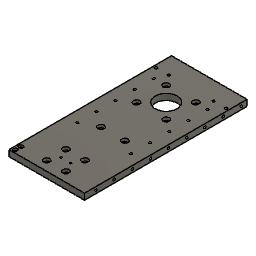
Z-AxisAssy v53 (Autodesk Fusion 360 archive; units mm, degrees)
design "PlaceHeadPlate" references "tormach 770mx"
Autodesk Fusion 360 part; units mm, degrees
sketch "Sketch1" plane through (0, 0, 0) normal (0, 1, 0) x (1, 0, 0)
  line L0 (0, 0) -> (79, 0)
  line L1 (79, 0) -> (79, -170)
  line L2 (79, -170) -> (0, -170)
  line L3 (0, -170) -> (0, 0)
  line L4 (39.5, 0) -> (39.5, -169.9926) construction
  line L5 (49.5, -160) -> (29.5, -160) construction
  line L6 (29.5, -160) -> (29.5, -140) construction
  line L7 (29.5, -140) -> (49.5, -140) construction
  line L8 (49.5, -140) -> (49.5, -160) construction
  line L9 (49.5, -160) -> (29.5, -140) construction
  line L10 (29.5, -160) -> (49.5, -140) construction
  line L11 (55, -60.5) -> (24, -60.5) construction
  line L12 (24, -60.5) -> (24, -29.5) construction
  line L13 (24, -29.5) -> (55, -29.5) construction
  line L14 (55, -29.5) -> (55, -60.5) construction
  line L15 (55, -60.5) -> (24, -29.5) construction
  line L16 (24, -60.5) -> (55, -29.5) construction
  circle A0 centre (39.5, -45) radius 11.5
  point P0 (67.5, -110)
  point P1 (11.5, -110)
  point P2 (67.5, -90)
  point P3 (11.5, -90)
  point P4 (67.5, -70)
  point P5 (11.5, -70)
  point P6 (67.5, -50)
  point P7 (11.5, -50)
  point P8 (67.5, -30)
  point P9 (11.5, -30)
  point P10 (39.5, -150)
  point P11 (29.5, -140)
  point P12 (49.5, -140)
  point P13 (49.5, -160)
  point P14 (29.5, -160)
  point P15 (44.5, -150)
  point P16 (34.5, -150)
  point P17 (3.5, -167)
  point P18 (3.5, -161)
  point P19 (27.58, -101.35)
  point P20 (52.58, -101.35)
  point P21 (39.5, -45)
  point P22 (24, -29.5)
  point P23 (55, -29.5)
  point P24 (55, -60.5)
  point P25 (24, -60.5)
  point P26 (16, -19)
  point P27 (63, -19)
  point P28 (2.86, -19)
  point P29 (76.14, -19)
  dimension "d1" = 79
  dimension "d2" = 170
  dimension "d5" = 60
  dimension "d6" = 11.5
  dimension "d7" = 56
  dimension "d10" = 0
  dimension "d11" = 20
  dimension "d15" = 20
  dimension "d16" = 20
  dimension "d17" = 10
  dimension "d18" = 10
  dimension "d19" = 5
  dimension "d20" = 6
  dimension "d21" = 3.5
  dimension "d22" = 3
  dimension "d23" = 25
  dimension "d24" = 68.65
  dimension "d25" = 11.92
  dimension "d26" = 31
  dimension "d27" = 31
  dimension "d28" = 29.5
  dimension "d29" = 24
  dimension "d31" = 16
  dimension "d32" = 16
  dimension "d33" = 19
  dimension "d34" = 13.14
  dimension "d35" = 13.14
  dimension "d36" = 19
  dimension "d42" = 23
  constraint horizontal L0
  constraint vertical L1
  constraint horizontal L2
  constraint vertical L3
  constraint coincident L0.start L3.end
  constraint horizontal P0 P1
  constraint perpendicular L2 L4
  constraint horizontal L5
  constraint perpendicular L5 L6
  constraint parallel L5 L7
  constraint parallel L6 L8
  constraint coincident L9 P10
  constraint coincident L10 P10
  constraint coincident L4 P10
  constraint coincident P11 L6.end
  constraint coincident P12 L7.end
  constraint coincident P13 L5.start
  constraint coincident P14 L5.end
  constraint horizontal P15 P16
  constraint vertical P17 P18
  constraint horizontal P19 P20
  constraint horizontal L11
  constraint perpendicular L11 L12
  constraint parallel L11 L13
  constraint parallel L12 L14
  constraint coincident L15 P21
  constraint coincident L16 P21
  constraint coincident L4 P21
  constraint coincident P22 L12.end
  constraint coincident P23 L13.end
  constraint coincident P24 L11.start
  constraint coincident P25 L11.end
  constraint horizontal P26 P27
  constraint horizontal P28 P29
  constraint coincident P21 A0.centre
  measures "d1" distance of L0.start L0.end
  measures "d2" distance of L0.start L2.end
  measures "d5" distance of L2 P0
  measures "d6" distance of L1 P0
  measures "d7" distance of P0 P1
  measures "d15" distance of P11 P12
  measures "d16" distance of L5 L7
  measures "d17" distance of L2 L5
  measures "d18" distance of P15 P16
  measures "d19" distance of L8 P15
  measures "d20" distance of P17 P18
  measures "d21" distance of L3 P17
  measures "d22" distance of L2 P17
  measures "d23" distance of P19 P20
  measures "d24" distance of L2 P19
  measures "d25" distance of L4 P19
  measures "d26" distance of P22 P23
  measures "d27" distance of P25 P22
  measures "d28" distance of L0 L13
  measures "d29" distance of L3 L12
  measures "d31" distance of L3 P26
  measures "d32" distance of L1 P27
  measures "d33" distance of L0 P26
  measures "d34" horizontal distance of P26 P28
  measures "d35" horizontal distance of P27 P29
  measures "d36" distance of L0 P28
  measures "d42" diameter of A0
extrude "Extrude2" add sketch "Sketch1" against normal blind 6.41
hole "Hole2" at (3.5, 0, 161) direction (0, -1, 0) diameter 2 end through all counterbore diameter 4.4 counterbore depth 2
hole "Hole3" at (3.5, 0, 167) direction (0, -1, 0) diameter 2 end through all counterbore diameter 4.4 counterbore depth 2
sketch "Sketch2" plane through (0, -6.41, 0) normal (0, -1, 0) x (1, 0, 0)
  circle A0 centre (3.5, 167) radius 1
  circle A1 centre (3.5, 161) radius 1
  circle A2 centre (39.5, 45) radius 11.5
  line L0 (79, 170) -> (0, 170)
  line L1 (0, 170) -> (0, 0)
  line L2 (0, 0) -> (79, 0)
  line L3 (79, 0) -> (79, 170)
  line L4 (49.5, 140) -> (49.5, 160)
  point P0 (44.5, 150)
  point P1 (34.5, 150)
  dimension "d55" = 5
  dimension "d56" = 10
  constraint horizontal P0 P1
  measures "d55" distance of P0 L4
  measures "d56" distance of P0 P1
hole "Hole4" at (34.5, -6.41, 150) direction (0, 1, 0) diameter 2 end through all counterbore diameter 4.4 counterbore depth 2
hole "Hole5" at (44.5, -6.41, 150) direction (0, 1, 0) diameter 2 end through all counterbore diameter 4.4 counterbore depth 2
hole "Hole6" at (29.5, 0, 140) direction (0, -1, 0) diameter 3.4 end through all counterbore diameter 6.5 counterbore depth 3
hole "Hole7" at (49.5, 0, 140) direction (0, -1, 0) diameter 3.4 end through all counterbore diameter 6.5 counterbore depth 3
hole "Hole8" at (29.5, 0, 160) direction (0, -1, 0) diameter 3.4 end through all counterbore diameter 6.5 counterbore depth 3
hole "Hole9" at (49.5, 0, 160) direction (0, -1, 0) diameter 3.4 end through all counterbore diameter 6.5 counterbore depth 3
hole "Hole10" at (27.58, 0, 101.35) direction (0, -1, 0) diameter 3.4 end through all counterbore diameter 6.5 counterbore depth 3
hole "Hole11" at (52.58, 0, 101.35) direction (0, -1, 0) diameter 3.4 end through all counterbore diameter 6.5 counterbore depth 3
hole "Hole12" at (24, 0, 29.5) direction (0, -1, 0) diameter 3.4 end through all counterbore diameter 6.5 counterbore depth 3
hole "Hole13" at (55, 0, 29.5) direction (0, -1, 0) diameter 3.4 end through all counterbore diameter 6.5 counterbore depth 3
hole "Hole14" at (55, 0, 60.5) direction (0, -1, 0) diameter 3.4 end through all counterbore diameter 6.5 counterbore depth 3
hole "Hole15" at (24, 0, 60.5) direction (0, -1, 0) diameter 3.4 end through all counterbore diameter 6.5 counterbore depth 3
hole "Hole16" at (11.5, 0, 110) direction (0, -1, 0) diameter 2.5 end through all
hole "Hole17" at (11.5, 0, 90) direction (0, -1, 0) diameter 2.5 end through all
hole "Hole18" at (11.5, 0, 70) direction (0, -1, 0) diameter 2.5 end through all
hole "Hole19" at (11.5, 0, 50) direction (0, -1, 0) diameter 2.5 end through all
hole "Hole20" at (11.5, 0, 30) direction (0, -1, 0) diameter 2.5 end through all
hole "Hole21" at (67.5, 0, 110) direction (0, -1, 0) diameter 2.5 end through all
hole "Hole22" at (67.5, 0, 90) direction (0, -1, 0) diameter 2.5 end through all
hole "Hole23" at (67.5, 0, 70) direction (0, -1, 0) diameter 2.5 end through all
hole "Hole24" at (67.5, 0, 50) direction (0, -1, 0) diameter 2.5 end through all
hole "Hole25" at (67.5, 0, 30) direction (0, -1, 0) diameter 2.5 end through all
hole "Hole26" at (16, 0, 19) direction (0, -1, 0) diameter 2.5 end through all
hole "Hole27" at (63, 0, 19) direction (0, -1, 0) diameter 2.5 end through all
hole "Hole28" at (2.86, 0, 19) direction (0, -1, 0) diameter 2.8 end through all
hole "Hole29" at (76.14, 0, 19) direction (0, -1, 0) diameter 2.8 end through all
sketch "TopHolesSketch" plane through (0, 0, 0) normal (0, 0, -1) x (-1, 0, 0)
  line L0 (0, 0) -> (-79, 0)
  line L1 (-79, 0) -> (-79, -6.41)
  line L2 (-79, -6.41) -> (0, -6.41)
  line L3 (0, -6.41) -> (0, 0)
  line L4 (0, -3.205) -> (-79, -3.205) construction
  point P0 (-14, -3.205)
  point P1 (-31, -3.205)
  point P2 (-48, -3.205)
  point P3 (-65, -3.205)
  dimension "d159" = 14
  dimension "d162" = -17
  dimension "d163" = 0
  constraint midpoint L3 L4.start
  constraint midpoint L1 L4.end
  constraint coincident L4 P0
  measures "d159" distance of L3 P0
hole "Hole30" at (14, -3.205, 0) direction (0, 0, 1) diameter 2.5 depth 10 tip angle 118
pattern_linear "R-Pattern1" count 4 spacing 17 along (1, 0, 0) of "Hole30"
sketch "Sketch4" plane through (0, 0, 0) normal (-1, 0, 0) x (0, 0, 1)
  line L0 (170, 0) -> (0, 0)
  line L1 (0, 0) -> (0, -6.41)
  line L2 (0, -6.41) -> (170, -6.41)
  line L3 (170, -6.41) -> (170, 0)
  line L4 (0, -3.205) -> (170, -3.205) construction
  point P0 (6, -3.205)
  point P1 (25, -3.205)
  point P2 (44, -3.205)
  point P3 (63, -3.205)
  point P4 (82, -3.205)
  point P5 (101, -3.205)
  point P6 (120, -3.205)
  point P7 (139, -3.205)
  point P8 (158, -3.205)
  dimension "d171" = 6
  dimension "d174" = 19
  dimension "d175" = 0
  constraint midpoint L1 L4.start
  constraint midpoint L3 L4.end
  constraint coincident L4 P0
  measures "d171" distance of L1 P0
sketch "Sketch5" plane through (79, 0, 0) normal (1, 0, 0) x (0, 0, -1)
  line L0 (0, 0) -> (-170, 0)
  line L1 (-170, 0) -> (-170, -6.41)
  line L2 (-170, -6.41) -> (0, -6.41)
  line L3 (0, -6.41) -> (0, 0)
  line L4 (0, -3.205) -> (-170, -3.205) construction
  point P0 (-6, -3.205)
  point P1 (-25, -3.205)
  point P2 (-44, -3.205)
  point P3 (-63, -3.205)
  point P4 (-82, -3.205)
  point P5 (-101, -3.205)
  point P6 (-120, -3.205)
  point P7 (-139, -3.205)
  point P8 (-158, -3.205)
  dimension "d176" = 6
  dimension "d179" = -19
  dimension "d180" = 0
  constraint midpoint L3 L4.start
  constraint midpoint L1 L4.end
  constraint coincident L4 P0
  measures "d176" distance of L3 P0
hole "Hole31" at (79, -3.205, 6) direction (-1, 0, 0) diameter 2.5 depth 10 tip angle 118
pattern_linear "R-Pattern2" count 1 spacing 19 along (0, -1, 0) count 9 spacing 19 along (0, 0, 1) of "Hole31"
hole "Hole32" at (0, -3.205, 6) direction (1, 0, 0) diameter 2.5 depth 10 tip angle 118
pattern_linear "R-Pattern3" count 1 spacing 0 along (0, -1, 0) count 9 spacing 19 along (0, 0, 1) of "Hole32"

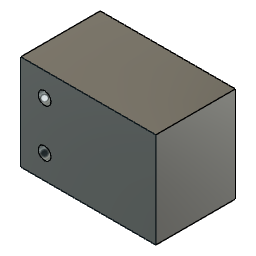
design "X-AxisLimitSwitchBlock"
Autodesk Fusion 360 part; units mm, degrees
sketch "Sketch1" plane through (0, 0, 0) normal (0, 1, 0) x (1, 0, 0)
  line L0 (0, 0) -> (17, 0)
  line L1 (17, 0) -> (17, -10)
  line L2 (17, -10) -> (0, -10)
  line L3 (0, -10) -> (0, 0)
  dimension "d1" = 17
  dimension "d2" = 10
  constraint horizontal L0
  constraint vertical L1
  constraint horizontal L2
  constraint vertical L3
  constraint coincident L0.start L3.end
  measures "d1" distance of L0.start L0.end
  measures "d2" distance of L0.start L2.end
extrude "Extrude1" add sketch "Sketch1" along normal blind 12
sketch "Sketch2" plane through (0, 0, 10) normal (0, 0, 1) x (1, 0, 0)
  line L0 (0, 0) -> (17, 0)
  line L1 (17, 0) -> (17, 12)
  line L2 (17, 12) -> (0, 12)
  line L3 (0, 12) -> (0, 0)
  point P0 (3, 3)
  point P1 (3, 9)
  dimension "d5" = 3
  dimension "d6" = 3
  dimension "d7" = 6
  measures "d5" distance of L0 P0
  measures "d6" distance of L3 P0
  measures "d7" distance of P0 P1
hole "Hole1" at (3, 3, 10) direction (0, 0, -1) diameter 1.6 depth 5 tip angle 118
hole "Hole2" at (3, 9, 10) direction (0, 0, -1) diameter 1.6 depth 5 tip angle 118

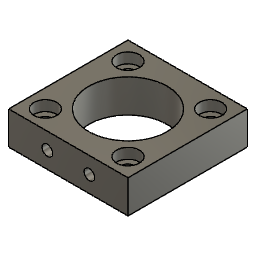
design "Nema8Mount" references "tormach 770mx"
Autodesk Fusion 360 part; units mm, degrees
sketch "Sketch1" plane through (0, 0, 0) normal (0, 1, 0) x (1, 0, 0)
  line L0 (11.55, -11.55) -> (-11.55, -11.55)
  line L1 (-11.55, -11.55) -> (-11.55, 11.55)
  line L2 (-11.55, 11.55) -> (11.55, 11.55)
  line L3 (11.55, 11.55) -> (11.55, -11.55)
  line L4 (11.55, -11.55) -> (-11.55, 11.55) construction
  line L5 (-11.55, -11.55) -> (11.55, 11.55) construction
  dimension "d1" = 23.1
  dimension "d2" = 23.1
  constraint horizontal L0
  constraint perpendicular L0 L1
  constraint parallel L0 L2
  constraint parallel L1 L3
  constraint coincident L4 origin
  constraint coincident L5 origin
  measures "d1" distance of L1.end L2.end
  measures "d2" distance of L0.end L1.end
extrude "Extrude1" add sketch "Sketch1" along normal blind 6.4
sketch "Sketch2" plane through (0, 6.4, 0) normal (0, 1, 0) x (-1, 0, 0)
  line L0 (-11.55, -11.55) -> (11.55, -11.55)
  line L1 (11.55, -11.55) -> (11.55, 11.55)
  line L2 (11.55, 11.55) -> (-11.55, 11.55)
  line L3 (-11.55, 11.55) -> (-11.55, -11.55)
  line L4 (-8, 8) -> (8, 8) construction
  line L5 (8, 8) -> (8, -8) construction
  line L6 (8, -8) -> (-8, -8) construction
  line L7 (-8, -8) -> (-8, 8) construction
  line L8 (-8, 8) -> (8, -8) construction
  line L9 (8, 8) -> (-8, -8) construction
  circle A0 centre (0, 0) radius 7.6
  point P0 (8, -8)
  point P1 (-8, -8)
  point P2 (-8, 8)
  point P3 (8, 8)
  dimension "d5" = 16
  dimension "d6" = 16
  dimension "d7" = 15.2
  constraint horizontal L4
  constraint perpendicular L4 L5
  constraint parallel L4 L6
  constraint parallel L5 L7
  constraint coincident L8 A0.centre
  constraint coincident L9 A0.centre
  constraint coincident A0.centre origin
  constraint coincident P0 L5.end
  constraint coincident P1 L6.end
  constraint coincident P2 L4.start
  constraint coincident P3 L4.end
  measures "d5" distance of P0 P1
  measures "d6" distance of P3 P0
  measures "d7" diameter of A0
hole "Hole1" at (-8, 6.4, -8) direction (0, -1, 0) diameter 2.2 end through all counterbore diameter 4.4 counterbore depth 2
hole "Hole2" at (8, 6.4, -8) direction (0, -1, 0) diameter 2.2 end through all counterbore diameter 4.4 counterbore depth 2
hole "Hole3" at (8, 6.4, 8) direction (0, -1, 0) diameter 2.2 end through all counterbore diameter 4.4 counterbore depth 2
hole "Hole4" at (-8, 6.4, 8) direction (0, -1, 0) diameter 2.2 end through all counterbore diameter 4.4 counterbore depth 2
extrude "Extrude2" cut sketch "Sketch2" along normal through all and the other way through all contours A0
sketch "Sketch3" plane through (0, 0, 11.55) normal (0, 0, 1) x (1, 0, 0)
  line L0 (-11.55, 0) -> (11.55, 0)
  line L1 (11.55, 0) -> (11.55, 6.4)
  line L2 (11.55, 6.4) -> (-11.55, 6.4)
  line L3 (-11.55, 6.4) -> (-11.55, 0)
  line L4 (-11.55, 3.2) -> (11.55, 3.2) construction
  point P0 (-4.15, 3.2)
  point P1 (3.99, 3.2)
  dimension "d29" = 8.14
  dimension "d30" = 7.4
  constraint midpoint L3 L4.start
  constraint midpoint L1 L4.end
  constraint coincident L4 P0
  constraint coincident L4 P1
  measures "d29" distance of P0 P1
  measures "d30" distance of L3 P0
hole "Hole5" at (-4.07, 3.2, 11.55) direction (0, 0, -1) diameter 2.05 depth 7 tip angle 118
hole "Hole6" at (4.07, 3.2, 11.55) direction (0, 0, -1) diameter 2.05 depth 7 tip angle 118

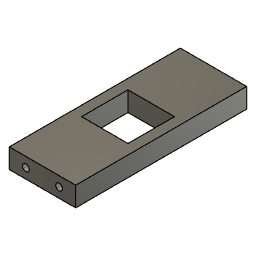
design "CameraHolder" references "tormach 770mx"
Autodesk Fusion 360 part; units mm, degrees
sketch "Sketch1" plane through (0, 0, 0) normal (0, 1, 0) x (1, 0, 0)
  line L0 (0, 0) -> (20, 0)
  line L1 (20, 0) -> (20, -51.54)
  line L2 (20, -51.54) -> (0, -51.54)
  line L3 (0, -51.54) -> (0, 0)
  dimension "d1" = 20
  dimension "d2" = 51.54
  constraint horizontal L0
  constraint vertical L1
  constraint horizontal L2
  constraint vertical L3
  constraint coincident L0.start L3.end
  measures "d1" distance of L0.start L0.end
  measures "d2" distance of L0.start L2.end
extrude "Extrude1" add sketch "Sketch1" along normal blind 5.92
sketch "Sketch2" plane through (0, 5.92, 0) normal (0, 1, 0) x (-1, 0, 0)
  line L0 (0, 51.54) -> (-20, 51.54)
  line L1 (-20, 51.54) -> (-20, 0)
  line L2 (-20, 0) -> (0, 0)
  line L3 (0, 0) -> (0, 51.54)
  line L4 (-10, 0) -> (-10, 49) construction
  line L5 (0, 25.77) -> (-20, 25.77) construction
  line L6 (-3, 32.77) -> (-17, 32.77)
  line L7 (-17, 32.77) -> (-17, 18.77)
  line L8 (-17, 18.77) -> (-3, 18.77)
  line L9 (-3, 18.77) -> (-3, 32.77)
  line L10 (-3, 32.77) -> (-17, 18.77) construction
  line L11 (-17, 32.77) -> (-3, 18.77) construction
  point P0 (-10, 25.77)
  dimension "d5" = 14
  dimension "d6" = 14
  constraint midpoint L2 L4.start
  constraint perpendicular L2 L4
  constraint midpoint L3 L5.start
  constraint midpoint L1 L5.end
  constraint horizontal L6
  constraint perpendicular L6 L7
  constraint parallel L6 L8
  constraint parallel L7 L9
  constraint coincident L10 P0
  constraint coincident L11 P0
  constraint midpoint L5 P0
  constraint coincident L9.start L8
  constraint coincident L8.end L9
  constraint coincident L7.end L8
  constraint coincident L8.start L7
  constraint coincident L6.start L9
  constraint coincident L9.end L6
  constraint coincident L6.end L7
  constraint coincident L7.start L6
  measures "d5" distance of L7.end L8.end
  measures "d6" distance of L6.end L7.end
extrude "Extrude2" cut sketch "Sketch2" along normal through all and the other way through all contours L6 L7 L8 L9
sketch "Sketch3" plane through (0, 0, 51.54) normal (0, 0, 1) x (1, 0, 0)
  line L0 (0, 0) -> (20, 0)
  line L1 (20, 0) -> (20, 5.92)
  line L2 (20, 5.92) -> (0, 5.92)
  line L3 (0, 5.92) -> (0, 0)
  line L4 (10, 5.92) -> (10, 0) construction
  line L5 (20, 2.96) -> (0, 2.96) construction
  point P0 (5, 2.96)
  point P1 (15, 2.96)
  dimension "d12" = 10
  dimension "d13" = 5
  constraint midpoint L2 L4.start
  constraint midpoint L0 L4.end
  constraint midpoint L1 L5.start
  constraint midpoint L3 L5.end
  constraint coincident L5 P0
  constraint coincident L5 P1
  measures "d12" distance of P0 P1
  measures "d13" distance of L5.end P0
hole "Hole1" at (5, 2.96, 51.54) direction (0, 0, -1) diameter 2.05 depth 10 tip angle 118
hole "Hole2" at (15, 2.96, 51.54) direction (0, 0, -1) diameter 2.05 depth 10 tip angle 118
sketch "Sketch4" plane through (0, 0, 0) normal (0, 0, -1) x (-1, 0, 0)
  line L0 (-20, 0) -> (0, 0)
  line L1 (0, 0) -> (0, 5.92)
  line L2 (0, 5.92) -> (-20, 5.92)
  line L3 (-20, 5.92) -> (-20, 0)
  line L4 (-20, 2.96) -> (0, 2.96) construction
  point P0 (-15, 2.96)
  point P1 (-5, 2.96)
  dimension "d30" = 10
  dimension "d31" = 5
  constraint midpoint L3 L4.start
  constraint midpoint L1 L4.end
  constraint coincident L4 P0
  constraint coincident L4 P1
  measures "d30" distance of P0 P1
  measures "d31" distance of L3 P0
hole "Hole5" at (15, 2.96, 0) direction (0, 0, 1) diameter 2.05 depth 10 tip angle 118
hole "Hole6" at (5, 2.96, 0) direction (0, 0, 1) diameter 2.05 depth 10 tip angle 118

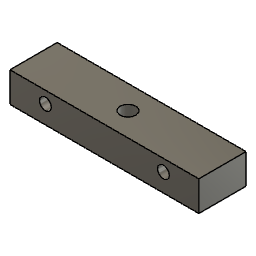
design "CableClampBracket" references "tormach 770mx"
Autodesk Fusion 360 part; units mm, degrees
sketch "Sketch1" plane through (0, 0, 0) normal (0, 1, 0) x (1, 0, 0)
  line L0 (0, 0) -> (40, 0)
  line L1 (40, 0) -> (40, -10)
  line L2 (40, -10) -> (0, -10)
  line L3 (0, -10) -> (0, 0)
  dimension "d1" = 40
  dimension "d2" = 10
  constraint horizontal L0
  constraint vertical L1
  constraint horizontal L2
  constraint vertical L3
  constraint coincident L0.start L3.end
  measures "d1" distance of L0.start L0.end
  measures "d2" distance of L0.start L2.end
extrude "Extrude1" add sketch "Sketch1" along normal blind 6.35
sketch "Sketch2" plane through (0, 6.35, 0) normal (0, 1, 0) x (-1, 0, 0)
  line L0 (0, 10) -> (-40, 10)
  line L1 (-40, 10) -> (-40, 0)
  line L2 (-40, 0) -> (0, 0)
  line L3 (0, 0) -> (0, 10)
  line L4 (0, 5) -> (-40, 5) construction
  point P0 (-20, 5)
  constraint midpoint L3 L4.start
  constraint midpoint L1 L4.end
  constraint midpoint L4 P0
hole "Hole1" at (20, 6.35, 5) direction (0, -1, 0) diameter 3.3 end through all
sketch "Sketch3" plane through (0, 0, 10) normal (0, 0, 1) x (1, 0, 0)
  line L0 (0, 0) -> (40, 0)
  line L1 (40, 0) -> (40, 6.35)
  line L2 (40, 6.35) -> (0, 6.35)
  line L3 (0, 6.35) -> (0, 0)
  line L4 (0, 3.85) -> (39.5878, 3.85) construction
  point P0 (7.5, 3.85)
  point P1 (32.5, 3.85)
  dimension "d10" = 7.5
  dimension "d11" = 25
  dimension "d18" = 2.5
  constraint coincident L4 P0
  constraint coincident L4 P1
  measures "d10" distance of L3 P0
  measures "d11" distance of P0 P1
  measures "d18" distance of L2 L4
hole "Hole4" at (7.5, 3.85, 10) direction (0, 0, -1) diameter 2.5 end through all
hole "Hole5" at (32.5, 3.85, 10) direction (0, 0, -1) diameter 2.5 end through all
hole "Hole2" [suppressed]
hole "Hole3" [suppressed]

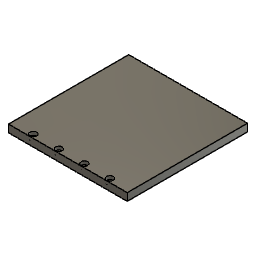
design "PlaceHeadCover"
Autodesk Fusion 360 part; units mm, degrees
sketch "Sketch1" plane through (0, 0, 0) normal (0, 1, 0) x (1, 0, 0)
  line L0 (0, 0) -> (79, 0)
  line L1 (79, 0) -> (79, -80)
  line L2 (79, -80) -> (0, -80)
  line L3 (0, -80) -> (0, 0)
  dimension "d1" = 79
  dimension "d2" = 80
  constraint horizontal L0
  constraint vertical L1
  constraint horizontal L2
  constraint vertical L3
  constraint coincident L0.start L3.end
  measures "d1" distance of L0.start L0.end
  measures "d2" distance of L0.start L2.end
extrude "Extrude1" add sketch "Sketch1" along normal blind 5
sketch "Sketch2" plane through (0, 5, 0) normal (0, 1, 0) x (-1, 0, 0)
  line L0 (0, 80) -> (-79, 80)
  line L1 (-79, 80) -> (-79, 0)
  line L2 (-79, 0) -> (0, 0)
  line L3 (0, 0) -> (0, 80)
  point P0 (-14, 77.5)
  dimension "d5" = 14
  dimension "d6" = 2.5
  measures "d5" distance of L3 P0
  measures "d6" distance of L0 P0
hole "Hole1" at (14, 5, 77.5) direction (0, -1, 0) diameter 2 end through all counterbore diameter 4.4 counterbore depth 2.2
pattern_linear "R-Pattern1" count 1 spacing 0 along (0, 0, -1) count 4 spacing 17 along (1, 0, 0) of "Hole1"

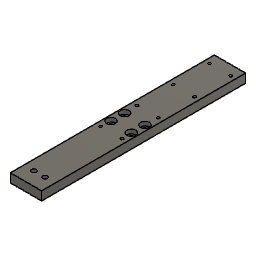
design "Z-AxisGearRackPlateFixed" references "tormach 770mx"
Autodesk Fusion 360 part; units mm, degrees
sketch "Sketch1" plane through (0, 0, 0) normal (0, 1, 0) x (1, 0, 0)
  line L0 (0, 0) -> (23, 0)
  line L1 (23, 0) -> (23, -150)
  line L2 (23, -150) -> (0, -150)
  line L3 (0, -150) -> (0, 0)
  dimension "d1" = 23
  dimension "d2" = 150
  constraint horizontal L0
  constraint vertical L1
  constraint horizontal L2
  constraint vertical L3
  constraint coincident L0.start L3.end
  measures "d1" distance of L0.start L0.end
  measures "d2" distance of L0.start L2.end
extrude "Extrude1" add sketch "Sketch1" along normal blind 6.43
sketch "Sketch2" plane through (0, 6.43, 0) normal (0, 1, 0) x (1, 0, 0)
  line L0 (11.5, 0) -> (11.5, -150) construction
  line L1 (0, 0) -> (0, -150)
  line L2 (0, -75) -> (23, -75) construction
  line L3 (19, -70) -> (4, -70) construction
  line L4 (4, -70) -> (4, -80) construction
  line L5 (4, -80) -> (19, -80) construction
  line L6 (19, -80) -> (19, -70) construction
  line L7 (19, -70) -> (4, -80) construction
  line L8 (4, -70) -> (19, -80) construction
  line L9 (23, 0) -> (0, 0)
  line L10 (0, -150) -> (23, -150)
  line L11 (0, -150) -> (23, -150)
  line L12 (23, -150) -> (23, 0)
  line L13 (23, 0) -> (0, 0)
  line L14 (0, 0) -> (0, -150)
  point P0 (11.5, -75)
  point P1 (4, -70)
  point P2 (19, -70)
  point P3 (19, -80)
  point P4 (4, -80)
  point P5 (3.7, -7.25)
  point P6 (19.3, -7.25)
  point P7 (3.7, -33.92)
  point P8 (3.7, -60.59)
  point P9 (3.7, -87.26)
  point P10 (19.3, -33.92)
  point P11 (19.3, -60.59)
  point P12 (19.3, -87.26)
  dimension "d5" = 11.5
  dimension "d6" = 15
  dimension "d7" = 10
  dimension "d8" = 15.6
  dimension "d9" = 19.3
  dimension "d10" = 7.25
  dimension "d13" = 0
  dimension "d14" = -26.67
  dimension "d17" = 0
  dimension "d18" = -26.67
  constraint vertical L0
  constraint midpoint L1 L2.start
  constraint perpendicular L0 L2
  constraint horizontal L3
  constraint perpendicular L3 L4
  constraint parallel L3 L5
  constraint parallel L4 L6
  constraint coincident L7 P0
  constraint coincident L8 P0
  constraint midpoint L0 P0
  constraint coincident P1 L3.end
  constraint coincident P2 L3.start
  constraint coincident P3 L5.end
  constraint coincident P4 L4.end
  constraint horizontal P5 P6
  measures "d5" distance of L0 L1
  measures "d6" distance of P4 P3
  measures "d7" distance of P1 P4
  measures "d8" distance of P5 P6
  measures "d9" distance of L1 P6
  measures "d10" distance of P5 L9
hole "Hole1" at (4, 6.43, 70) direction (0, -1, 0) diameter 3.4 end through all counterbore diameter 6.5 counterbore depth 3
hole "Hole2" at (19, 6.43, 70) direction (0, -1, 0) diameter 3.4 end through all counterbore diameter 6.5 counterbore depth 3
hole "Hole3" at (4, 6.43, 80) direction (0, -1, 0) diameter 3.4 end through all counterbore diameter 6.5 counterbore depth 3
hole "Hole4" at (19, 6.43, 80) direction (0, -1, 0) diameter 3.4 end through all counterbore diameter 6.5 counterbore depth 3
hole "Hole5" at (3.7, 6.43, 7.25) direction (0, -1, 0) diameter 2.05 end through all
hole "Hole6" at (19.3, 6.43, 7.25) direction (0, -1, 0) diameter 2.05 end through all
hole "Hole7" at (3.7, 6.43, 33.92) direction (0, -1, 0) diameter 2.05 end through all
hole "Hole8" at (19.3, 6.43, 33.92) direction (0, -1, 0) diameter 2.05 end through all
hole "Hole9" at (3.7, 6.43, 60.59) direction (0, -1, 0) diameter 2.05 end through all
hole "Hole10" at (19.3, 6.43, 60.59) direction (0, -1, 0) diameter 2.05 end through all
hole "Hole11" at (3.7, 6.43, 87.26) direction (0, -1, 0) diameter 2.05 end through all
hole "Hole12" at (19.3, 6.43, 87.26) direction (0, -1, 0) diameter 2.05 end through all
sketch "Sketch3" plane through (0, 0, 0) normal (0, -1, 0) x (1, 0, 0)
  circle A0 centre (19.3, 87.26) radius 1.025
  circle A1 centre (3.7, 87.26) radius 1.025
  circle A2 centre (19.3, 60.59) radius 1.025
  circle A3 centre (3.7, 60.59) radius 1.025
  circle A4 centre (19.3, 33.92) radius 1.025
  circle A5 centre (3.7, 33.92) radius 1.025
  circle A6 centre (19.3, 7.25) radius 1.025
  circle A7 centre (3.7, 7.25) radius 1.025
  circle A8 centre (19, 80) radius 1.7
  circle A9 centre (4, 80) radius 1.7
  circle A10 centre (19, 70) radius 1.7
  circle A11 centre (4, 70) radius 1.7
  line L0 (23, 150) -> (0, 150)
  line L1 (0, 150) -> (0, 0)
  line L2 (0, 0) -> (23, 0)
  line L3 (23, 0) -> (23, 150)
  line L4 (0, 150) -> (23, 150)
  point P0 (15.6, 140)
  point P1 (7.46, 140)
  dimension "d92" = 8.14
  dimension "d93" = 10
  dimension "d94" = 7.4
  constraint horizontal P0 P1
  measures "d92" distance of P0 P1
  measures "d93" distance of P0 L4
  measures "d94" distance of L3 P0
hole "Hole17" at (7.4, 0, 140) direction (0, 1, 0) diameter 3.4 end through all counterbore diameter 6.5 counterbore depth 3
hole "Hole18" at (15.54, 0, 140) direction (0, 1, 0) diameter 3.4 end through all counterbore diameter 6.5 counterbore depth 3
